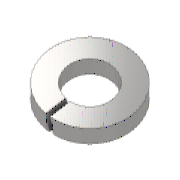
# Autodesk Inventor part: SpringWasher_M3-0.7
Saved by Autodesk Inventor 2024 (Build 280153000, 153)
## iProperties
Created: 2022-10-16
Part Number: SpringWasher_M3-0.7
Material: 鋼、軟鋼
Description: スプリングワッシャー
Document SubType Name: Modeling
Designer: jwith
Manufacturer: Y.H.
Language: ja-JP
Size Designation: M3-1.1
Categories: <MemberInstance><Categories><Category DisplayName="締結器具" InternalName="e4da775c-781d-43d5-af7c-5136215cf5a6" Mnemonic="FSTN"><Category DisplayName="座金" InternalName="337c07a8-832c-4473-9e51-3c1dc967456d" Mnemonic="WSHR"><CategoryParameter DisplayName="ボルトの直径" InternalName="5ec4e49b-d828-412c-aba4-3e4311d0c7bd" Mnemonic="bltdia"/><CategoryParameter DisplayName="厚さ" InternalName="e5901bd4-d58f-484f-966d-ad4eee01a60f" Mnemonic="wthick"/><Category DisplayName="ばね" InternalName="0d23ad87-adc1-46e2-86d3-ffd77355fdb5" Mnemonic="SPLWASH"><CategoryParameter DisplayName="タイプ" InternalName="3d847ff2-8ea8-43db-954e-352837e6dc30" Mnemonic="type"/><CategoryParameter DisplayName="外径" InternalName="e60beade-987e-4bc0-94d8-bcfc528051e4" Mnemonic="woutdia"/></Category></Category></Category><Category DisplayName="データタイプ" InternalName="23b78d0f-2648-40c6-8793-ca6db495c9e8" Mnemonic="DATATYPE"><CategoryParameter DisplayName="表示名" InternalName="05415f3d-3907-474b-a020-eb9d644f4cf3" Mnemonic="DISPLAYNAME"/><CategoryParameter DisplayName="規格" InternalName="0c0a119c-1e12-4c84-803f-101930972f5e" Mnemonic="STANDARD"/><CategoryParameter DisplayName="説明" InternalName="13903e3d-64b1-4950-80da-f627842ea37f" Mnemonic="DESCRIPTION"/><CategoryParameter DisplayName="指定" InternalName="2675968c-4ce5-49e0-a4f5-552d29089031" Mnemonic="DESIGNATION"/><CategoryParameter DisplayName="既定行" InternalName="2af9ec52-faaa-4026-b378-f9fa4afca842" Mnemonic="DEFAULTROW"/><CategoryParameter DisplayName="フォルダ名" InternalName="3f06958e-8713-4116-9be7-ed6184ecc97b" Mnemonic="FOLDERNAME"/><CategoryParameter DisplayName="リビジョン ガイド" InternalName="45a75005-10b1-4dfc-8d6d-dfe629f0b93c" Mnemonic="REVISIONGUID"/><CategoryParameter DisplayName="ファイル名" InternalName="8b46a4cc-9585-4fed-90c3-899f57e09a73" Mnemonic="FILENAME"/><CategoryParameter DisplayName="標準化団体" InternalName="8f5914e1-4693-403f-8ab5-d37768198c9d" Mnemonic="STDSORG"/><CategoryParameter DisplayName="ファミリ バージョン" InternalName="914462f6-6e19-4b14-ba84-155b9680b1d0" Mnemonic="FAMILYREVISION"/><CategoryParameter DisplayName="規格のリビジョン" InternalName="91d5a463-65c2-4fde-b823-3b7fea5e8e17" Mnemonic="STANDARDREVISION"/><CategoryParameter DisplayName="メンバ履歴" InternalName="a65d44b9-392f-4f4f-857b-e4b3d54996fe" Mnemonic="MEMBERREVISION"/><CategoryParameter DisplayName="クリップ フォーマット" InternalName="bc51e27b-3422-4e78-93ef-cec197ddf230" Mnemonic="CLIPFORMAT"/><CategoryParameter DisplayName="製造者" InternalName="cd6c7a72-a28a-4e50-99a9-2c7f4e13e5ad" Mnemonic="MANUFACTURER"/><CategoryParameter DisplayName="内部名" InternalName="cf1d0246-76d9-4b4a-8305-fa0409afb5c1" Mnemonic="INTERNALNAME"/><CategoryParameter DisplayName="IsMetric" InternalName="e2385c5b-1ea4-4823-96a8-8de651266ec3" Mnemonic="ISMETRIC"/><Category DisplayName="パーツ" InternalName="c0e0b642-3bcb-4cc8-9e80-f96d35c4afa4" Mnemonic="PART"><CategoryParameter DisplayName="部品番号" InternalName="016b6077-bfbe-49bd-92c9-d8d59c39c941" Mnemonic="PARTNUMBER"/><CategoryParameter DisplayName="ストック番号" InternalName="4dba7c1c-e26c-444e-836c-b08b433409a8" Mnemonic="STOCKNUMBER"/><CategoryParameter DisplayName="材料キー" InternalName="5c9a8adb-dd2b-4535-b97f-0a94a95fe41f" Mnemonic="MATERIALKEY"/><CategoryParameter DisplayName="材料" InternalName="818a152a-d3c3-49ca-80ee-df7d91421b8e" Mnemonic="MATERIAL"/></Category></Category></Categories><FamilyTemplate Id="SpringWasher"><FamilyTemplateParameters><FamilyTemplateParameter ObjectType="kUserParameterObject" ValueType="xs:double" Id="31" ObjectReferenceKey="NominalDiam"/><FamilyTemplateParameter ObjectType="kUserParameterObject" ValueType="xs:double" Id="32" ObjectReferenceKey="Thick"/><FamilyTemplateParameter ObjectType="kUserParameterObject" ValueType="xs:double" Id="33" ObjectReferenceKey="OuterDiam"/><FamilyTemplateParameter ObjectType="kUserParameterObject" ValueType="xs:double" Id="54" ObjectReferenceKey="Height"/><FamilyTemplateParameter ObjectType="kUserParameterObject" ValueType="xs:double" Id="55" ObjectReferenceKey="InnerDiam"/><FamilyTemplateParameter ObjectType="kPartComponentDefinitionObject" ValueType="xs:string" Id="44" SubObjectId="Material"/><FamilyTemplateParameter ObjectType="kPropertyObject" ValueType="xs:string" Id="50" ObjectReferenceKey="{32853F0F-3444-11d1-9E93-0060B03C1CA6}" SubObjectId="5"/><FamilyTemplateParameter ObjectType="kRenderStyleObject" ValueType="xs:string" Id="52" SubObjectId="RenderStyle"/><FamilyTemplateParameter ObjectType="kPropertyObject" ValueType="xs:string" Id="57" ObjectReferenceKey="{D5CDD505-2E9C-101B-9397-08002B2CF9AE}" SubObjectId="Type"/></FamilyTemplateParameters></FamilyTemplate><CategoryParameterMap><ParamToTemplateMap><ParamToTemplate CategoryParameter="//CategoryParameter[@InternalName='cf1d0246-76d9-4b4a-8305-fa0409afb5c1']" ConstantValue="51a31c71-737f-4fbe-b8b1-0ed19b17a103"/><ParamToTemplate CategoryParameter="//CategoryParameter[@InternalName='45a75005-10b1-4dfc-8d6d-dfe629f0b93c']" ConstantValue="c5a52bea-ffaa-44eb-bbcd-1a899d499c21"/><ParamToTemplate CategoryParameter="//CategoryParameter[@InternalName='3f06958e-8713-4116-9be7-ed6184ecc97b']" ConstantValue="SpringWasher"/><ParamToTemplate CategoryParameter="//CategoryParameter[@InternalName='8f5914e1-4693-403f-8ab5-d37768198c9d']" TemplateParameter="38"/><ParamToTemplate CategoryParameter="//CategoryParameter[@InternalName='0c0a119c-1e12-4c84-803f-101930972f5e']" TemplateParameter="39"/><ParamToTemplate CategoryParameter="//CategoryParameter[@InternalName='91d5a463-65c2-4fde-b823-3b7fea5e8e17']" TemplateParameter="40"/><ParamToTemplate CategoryParameter="//CategoryParameter[@InternalName='cd6c7a72-a28a-4e50-99a9-2c7f4e13e5ad']" ConstantValue="Y.H."/><ParamToTemplate CategoryParameter="//CategoryParameter[@InternalName='13903e3d-64b1-4950-80da-f627842ea37f']" ConstantValue="スプリングワッシャー"/><ParamToTemplate CategoryParameter="//CategoryParameter[@InternalName='05415f3d-3907-474b-a020-eb9d644f4cf3']" ConstantValue="SpringWasher"/><ParamToTemplate CategoryParameter="//CategoryParameter[@InternalName='914462f6-6e19-4b14-ba84-155b9680b1d0']" ConstantValue="11"/><ParamToTemplate CategoryParameter="//CategoryParameter[@InternalName='bc51e27b-3422-4e78-93ef-cec197ddf230']" ConstantValue="CF_INVENTOR.STDPARTS"/><ParamToTemplate CategoryParameter="//CategoryParameter[@InternalName='e2385c5b-1ea4-4823-96a8-8de651266ec3']" ConstantValue="true"/><ParamToTemplate CategoryParameter="//CategoryParameter[@InternalName='2af9ec52-faaa-4026-b378-f9fa4afca842']" ConstantValue="1"/><ParamToTemplate CategoryParameter="//CategoryParameter[@InternalName='8b46a4cc-9585-4fed-90c3-899f57e09a73']" ConstantValue="SpringWasher_3007SL"/><ParamToTemplate CategoryParameter="//CategoryParameter[@InternalName='2675968c-4ce5-49e0-a4f5-552d29089031']" ConstantValue="M3-1.1"/><ParamToTemplate CategoryParameter="//CategoryParameter[@InternalName='a65d44b9-392f-4f4f-857b-e4b3d54996fe']" ConstantValue="b048ca5b-82f7-4ba7-8eb6-d0e9e15c9cb2"/><ParamToTemplate CategoryParameter="//CategoryParameter[@InternalName='a65d44b9-392f-4f4f-857b-e4b3d54996fe']" ConstantValue="b048ca5b-82f7-4ba7-8eb6-d0e9e15c9cb2"/><ParamToTemplate CategoryParameter="//CategoryParameter[@InternalName='818a152a-d3c3-49ca-80ee-df7d91421b8e']" TemplateParameter="44"/><ParamToTemplate CategoryParameter="//CategoryParameter[@InternalName='5ec4e49b-d828-412c-aba4-3e4311d0c7bd']" TemplateParameter="31"/><ParamToTemplate CategoryParameter="//CategoryParameter[@InternalName='e60beade-987e-4bc0-94d8-bcfc528051e4']" TemplateParameter="33"/><ParamToTemplate CategoryParameter="//CategoryParameter[@InternalName='016b6077-bfbe-49bd-92c9-d8d59c39c941']" TemplateParameter="50"/><ParamToTemplate CategoryParameter="//CategoryParameter[@InternalName='e5901bd4-d58f-484f-966d-ad4eee01a60f']" TemplateParameter="32"/></ParamToTemplateMap></CategoryParameterMap></MemberInstance>
Density: 7.85 g/cm^3
Appearance: 半つや出し
Type: SpringWasher
IsCustomPart: 0
Author: jwith
Autodesk Inventor part; units mm, degrees
ref_plane "YZ Plane" through (0, 0, 0) normal (1, 0, 0) x (0, 1, 0)
ref_plane "XY Plane" through (0, 0, 0) normal (0, 0, 1) x (1, 0, 0)
sketch "スケッチ1" plane through (0, 0, 0) normal (0, 0, 1) x (0, 1, 0)
  circle A0 centre (0, 0) radius 1.55
  circle A1 centre (0, 0) radius 2.95
  dimension "d0" = 3.1
  dimension "d1" = 5.9
  constraints: 2 centre point, 2 coincident
  measures "d0" diameter of A0
  measures "d1" diameter of A1
extrude "ボディ" add sketch "スケッチ1" along normal blind 0.7
sketch "スケッチ2" plane through (0, 0, 0) normal (1, 0, 0) x (0, 0, -1)
  line L0 (0, 2.95) -> (0, -2.95) projected
  line L1 (-0.7, 2.95) -> (-0.7, -2.95) projected
  line L2 (-0.7, 0) -> (0, 0) construction
  line L3 (-0.7, 0.14) -> (0, 0.3948)
  line L4 (-0.7, -0.14) -> (0, 0.1148)
  line L5 (0.1, 0) -> (-0.6, 0) projected
  dimension "d4" = 0.14
  dimension "d5" = 0.14
  dimension "d6" = 70
  constraints: 6 end point, 4 point on line, 2 midpoint, 1 collinear, 1 parallel
  measures "d4" distance from line of L3.start L2
  measures "d5" distance from line of L4.start L2
  measures "d6" angle of L0 L3
extrude "切断" cut sketch "スケッチ2" along normal through all contours L0 L4 L1 L3
ref_plane "作業平面1" through (0, 0, 0) normal (0, 1, 0) x (-1, 0, 0)
equation "\"d0\" = InnerDiam"
equation "\"d1\" = OuterDiam"
equation "\"d2\" = Height"
equation "\"d4\" = 0.2 * Height"
equation "\"d5\" = 0.2 * Height"
equation "\"d6\" = ChamferAngle"
equation "\"InnerDiam\" = 3.1"
equation "\"OuterDiam\" = 5.9"
equation "\"Height\" = 0.7"
equation "\"ChamferAngle\" = 70deg"
equation "\"Thick\" = 1.1"
equation "\"NominalDiam\" = 3"
